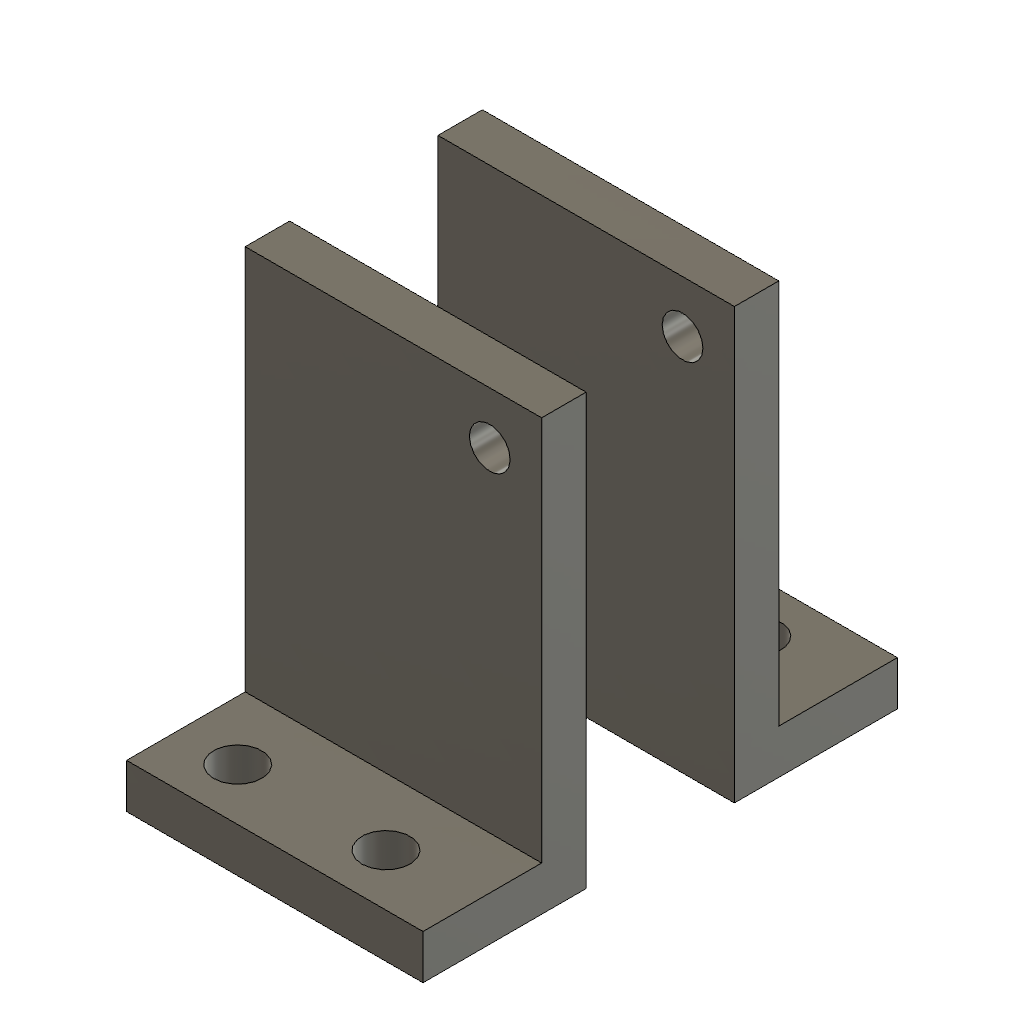
TankBot Bumper Switch Mount (Autodesk Fusion 360 design; units mm, degrees)
Autodesk Fusion 360 part; units mm, degrees
box "BoxPrimitive1" add length 18 width 20 height 10 placed x (0, 0, 1) y (1, 0, 0) z (0, 1, 0) at (0, 0, 0)
box "BoxPrimitive2" add length 10 width 10 height 1 placed x (0, -1, 0) y (0, 0, -1) z (1, 0, 0) at (20, 10, 13)
extrude "Extrude1" add 1 faces at (20.3333, 3.3333, 13) along direction (0, 0, 1) blind 1
extrude "Extrude2" cut 1 faces at (20.3333, 3.3333, 3) along direction (0, 0, 1) blind 1
extrude "Extrude3" cut 1 faces at (21, 6.6667, 7.3333) along direction (-1, 0, 0) blind 17
extrude "Extrude4" cut 1 faces at (6.6667, 3.3333, 18) along direction (0, 0, -1) blind 1
extrude "Extrude5" cut 1 faces at (6.6667, 3.3333, 0) along direction (0, 0, 1) blind 1
box "BoxPrimitive3" add length 3 width 20 height 4.5 placed x (0, 1, 0) y (-1, 0, 0) z (0, 0, 1) at (20, 0, 17)
box "BoxPrimitive4" add length 3 width 20 height 4.5 placed x (0, 1, 0) y (1, 0, 0) z (0, 0, -1) at (0, 0, 1)
extrude "Extrude6" add 1 faces at (6.6667, 1, 21.5) along direction (0, 0, 1) blind 2.5
extrude "Extrude7" add 1 faces at (13.3333, 1, -3.5) along direction (0, 0, -1) blind 2.5
hole "Hole1" at (15, 3, -3.5) direction (0, -1, 0) diameter 3.25 depth 3 tip angle 180
extrude "Extrude8" add 1 faces at (13.3333, 1, -6) along direction (0, 0, -1) blind 1
hole "Hole2" at (5, 3, -3.5) direction (0, -1, 0) diameter 3.25 depth 3 tip angle 180
hole "Hole3" at (5, 3, 21.5) direction (0, -1, 0) diameter 3.25 depth 3 tip angle 180
hole "Hole4" at (15, 3, 21.5) direction (0, -1, 0) diameter 3.25 depth 3 tip angle 180
extrude "Extrude9" add 1 faces at (6.6667, 1, 24) along direction (0, 0, 1) blind 1
box "BoxPrimitive5" add length 3 width 20 height 18 placed x (0, 0, -1) y (-1, 0, 0) z (0, 1, 0) at (20, 10, 17)
box "BoxPrimitive6" add length 3 width 20 height 18 placed x (0, 0, -1) y (-1, 0, 0) z (0, 1, 0) at (20, 10, 4)
hole "Hole5" at (17.5, 25.5, 17) direction (0, 0, -1) diameter 2.75 depth 16 tip angle 180
extrude "Extrude10" cut 1 faces at (0, 5.3333, 7.3333) along direction (1, 0, 0) blind 1
extrude "Extrude11" add 1 faces at (20, 13.6667, 16) along direction (1, 0, 0) blind 1
extrude "Extrude12" add 1 faces at (20, 12.6667, 3) along direction (1, 0, 0) blind 1
extrude "Extrude13" add 1 faces at (7.6667, 28, 16) along direction (0, 1, 0) blind 1
extrude "Extrude14" add 1 faces at (7.6667, 28, 3) along direction (0, 1, 0) blind 1
